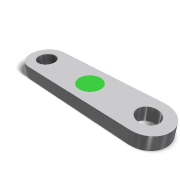
# Autodesk Inventor part: MI-2A003
Saved by Autodesk Inventor 2016 (Build 200138000, 138)
## iProperties
Created: 2012-01-08
Part Number: MI-2A003
Material: Generic
Document SubType Name: Modeling
Designer: Curtis
Density: 1 g/cm^3
Description: Hardware, Oblong Link
Appearance: Chrome - Polished Black
Author: Curtis
Autodesk Inventor part; units mm, degrees
ref_plane "YZ Plane" through (0, 0, 0) normal (1, 0, 0) x (0, 1, 0)
ref_plane "XZ Plane" through (0, 0, 0) normal (0, 1, 0) x (-1, 0, 0)
ref_plane "XY Plane" through (0, 0, 0) normal (0, 0, 1) x (1, 0, 0)
sketch "Sketch1" plane through (0, 0, 0) normal (0, 0, 1) x (1, 0, 0)
  line L0 (57.5, 15) -> (-57.5, 15)
  line L1 (-57.5, 15) -> (-57.5, -15)
  line L2 (-57.5, -15) -> (57.5, -15)
  line L3 (57.5, -15) -> (57.5, 15)
  line L4 (57.5, 15) -> (-57.5, -15) construction
  line L5 (-57.5, 15) -> (57.5, -15) construction
  point P0 (0, 0)
  dimension "d0" = 115
  dimension "d1" = 30
  constraints: 12 end point, 2 midpoint, 2 parallel, 1 horizontal, 1 perpendicular
  measures "d0" distance of L2.end L1.end
  measures "d1" distance of L1.end L0.end
extrude "Extrusion1" add sketch "Sketch1" along normal blind 10
full round fillet "Fillet1" first side at (-19.1667, -15, 6.6667) centre faces at (57.5, -5, 3.3333) second side at (19.1667, 15, 6.6667)
full round fillet "Fillet2" first side at (-24.1666, -15, 3.3333) centre faces at (-57.5, 5, 3.3333) second side at (9.1667, 15, 3.3333)
hole "Hole1" at (-42.5, 0, 10) direction (0, 0, -1) diameter 15 end through all
hole "Hole2" at (42.5, 0, 10) direction (0, 0, -1) diameter 15 end through all
sketch "Sketch2" plane through (0, 0, 10) normal (0, 0, 1) x (1, 0, 0)
  circle A0 centre (0, 0) radius 9
  dimension "d24" = 18
  constraints: 1 centre point, 1 coincident
  measures "d24" diameter of A0
split_face "Split1"
body "Solid1"
